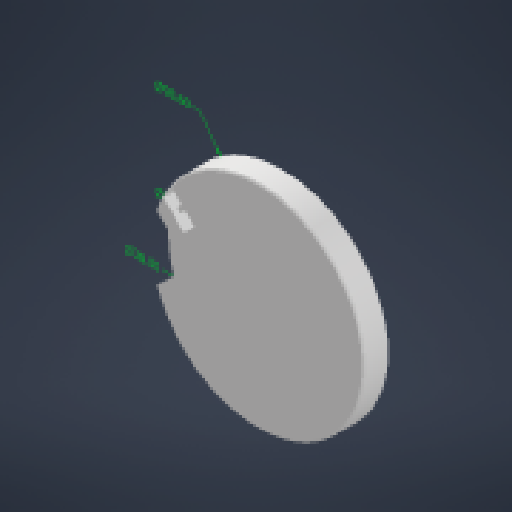
# Autodesk Inventor part: FlyCutter
Saved by Autodesk Inventor 2024.2 (Build 282272000, 272)
## iProperties
Created: 2024-03-09
Part Number: FlyCutter
Material: Generic
Document SubType Name: Modeling
Designer: LightStore
Density: 1 g/cm^3
Appearance: Default
Author: LightStore
Autodesk Inventor part; units mm, degrees
ref_plane "YZ Plane" through (0, 0, 0) normal (1, 0, 0) x (0, 1, 0)
ref_plane "XZ Plane" through (0, 0, 0) normal (0, 1, 0) x (-1, 0, 0)
ref_plane "XY Plane" through (0, 0, 0) normal (0, 0, 1) x (1, 0, 0)
sketch "Sketch1" plane through (0, 0, 0) normal (0, 0, 1) x (1, 0, 0)
  circle A0 centre (0, 0) radius 50
  dimension "d0" = 100
  constraints: 1 centre point, 1 coincident
  measures "d0" diameter of A0
extrude "Extrusion1" add sketch "Sketch1" along normal blind 12
sketch "Sketch2" plane through (0, 0, 0) normal (0, 0, -1) x (-1, 0, 0)
  circle A0 centre (0, 0) radius 15
  dimension "d3" = 30
  constraints: 1 centre point, 1 coincident
  measures "d3" diameter of A0
extrude "Extrusion2" add sketch "Sketch2" along normal blind 12
chamfer "Chamfer1" distance 0.7 angle 45 1 edges at (-50, 0, 0)
chamfer "Chamfer2" distance 0.7 angle 45 1 edges at (-50, 0, 12)
sketch "Sketch9" plane through (0, 0, -12) normal (0, 0, -1) x (-1, 0, 0)
  circle A0 centre (0, 0) radius 6
  circle A1 centre (0, 0) radius 4
  dimension "d32" = 12
  dimension "d33" = 8
  constraints: 2 centre point, 2 coincident
  measures "d32" diameter of A0
  measures "d33" diameter of A1
extrude "Extrusion9" add sketch "Sketch9" along normal blind 12
sketch "Sketch10" plane through (0, 0, 12) normal (0, 0, 1) x (1, 0, 0)
  circle A0 centre (0, 0) radius 49.3 projected
  line L0 (-46.9792, -14.9479) -> (-32.0415, 0)
  line L1 (-32.0415, 0) -> (-34.8474, 0)
  line L2 (-46.9792, 14.9479) -> (-32.0415, 0)
  line L3 (-46.9792, -14.9479) -> (-50.9309, -18.8996)
  line L4 (-46.9792, -14.9479) -> (-41.3907, -14.9479) construction
  line L5 (-46.9792, 14.9479) -> (-50.9309, 18.8996)
  arc A1 (-50.9309, 18.8996) -> (-50.9309, -18.8996) centre (-5.1445, 0) ccw
  arc A2 (-46.9792, 14.9479) -> (-46.9792, -14.9479) centre (0, 0) ccw
  line L6 (-17.4257, 0) -> (-43.6281, 26.2024)
  line L7 (-17.4257, 0) -> (19.6301, 0) construction
  line L8 (-12.476, 4.9497) -> (-38.6784, 31.1522)
  line L9 (-17.4257, 0) -> (-12.476, 4.9497)
  arc A3 (-38.4198, 30.8935) -> (-42.4668, 25.0411) centre (0, 0) ccw
  arc A4 (-38.6784, 31.1522) -> (-43.6281, 26.2024) centre (-36.0468, 23.5708) ccw
  dimension "d36" = 135
  dimension "d39" = 135
  constraints: 20 end point, 11 point on circle, 4 centre point, 3 horizontal, 2 concentric, 2 equal length, 2 symmetric about line, 1 perpendicular, 1 point on line
  measures "d36" angle of L3 L4
  measures "d39" angle of L7 L6
extrude "Extrusion10" cut sketch "Sketch10" against normal blind 8 contours L3 A1 L5 A0 | A0 L2 L0
sketch "Sketch11" plane through (0, 0, 12) normal (0, 0, 1) x (1, 0, 0)
  line L0 (-46.9792, 14.9479) -> (-32.0415, 0) projected
  line L1 (-39.5104, 7.474) -> (-34.5589, 12.422)
  line L2 (-22.1379, 0.0075) -> (-44.1228, 21.9924)
  circle A0 centre (0, 0) radius 49.3 projected
  line L3 (-34.5589, 12.422) -> (-29.6092, 17.3718)
  line L4 (-34.5589, 12.422) -> (-27.5589, 12.422) construction
  line L5 (-32.0841, 14.8969) -> (-29.6092, 12.422)
  line L6 (-17.1946, 4.9507) -> (-39.1796, 26.9357)
  line L7 (-22.1379, 0.0075) -> (-17.1946, 4.9507)
  line L8 (-39.1796, 26.9357) -> (-40.4406, 28.1966)
  line L9 (-44.1228, 21.9924) -> (-46.2441, 24.1138)
  line L10 (-40.4406, 28.1966) -> (-42.3953, 30.4724)
  arc A1 (-42.3953, 30.4724) -> (-46.289, 24.1586) centre (-36.8863, 22.7176) ccw
  arc A2 (-46.9792, -14.9479) -> (-46.9792, 14.9479) centre (0, 0) ccw projected
  point P0 (-34.5557, 12.4253)
  point P1 (-29.6124, 17.3685)
  dimension "d42" = 7
  dimension "d43" = 7
  dimension "d45" = 3
  dimension "d46" = 3
  constraints: 20 end point, 5 point on circle, 2 midpoint, 2 point on line, 2 symmetric about line, 1 centre point, 1 equal length, 1 horizontal, 1 parallel, 1 perpendicular
  measures "d42" distance of L1.start L1.end
  measures "d43" distance of L1.end L3.end
  measures "d45" distance of L2.end L9.end
  measures "d46" distance of L8.end L10.end
extrude "Extrusion11" cut sketch "Sketch11" against normal blind 8 contours A0 L8 L6 L3 L2
sketch "Sketch12" plane through (-46.9792, 14.9479, 4) normal (-0.7073, -0.7069, 0) x (0, 0, 1)
  circle A0 centre (3.8047, -3.4144) radius 1.5
  point P0 (-4, -43.7814)
  dimension "d49" = 3
  constraints: 1 centre point
  measures "d49" diameter of A0
extrude "Extrusion12" cut sketch "Sketch12" against normal blind 8
body "Solid1"
